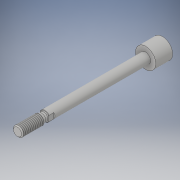
# Autodesk Inventor part: 8112003 DSNU-S-12-30-P---(P)
Saved by Autodesk Inventor 2019 (Build 230136000, 136)
## iProperties
Created: 2023-03-28
Part Number: 8112003 DSNU-S-12-30-P---(P)
Material: Generic
Catalog Web Link: www.cadenas.de
Description: DSNU-S---(P)-ISO cylinder
Vendor: FESTO
Document SubType Name: Modeling
Designer: psAdmin
Manufacturer: FESTO
Mass: 3.24458 g
Surface Area: 20.2529 cm^2
Volume: 3.24458 cm^3
Density: 1 g/cm^3
Appearance: PSOLRGB-175-175-175
Category: PARTsolutions
Company: FESTO
Title: 8112003 DSNU-S-12-30-P
Author: Cadenas PARTsolutions
Comments: ISO cylinder
PSOL_IDENT_0: {$CADENAS_DATA/23d-libs/festo/parts/d/dsnu/parts/dsnu_s_piston.prj},208 {VTYP=3D},{NB=8112003 DSNU-S
PSOL_IDENT_1: -12-30-P---(P)},{LINA=8112003 DSNU-S-12-30-P},{NN=DSNU-S---(P)},{DATE=13.03.2023 13:59:39},{GEOMDATE=
PSOL_IDENT_2: 01.06.2021 09:47:00},{VERSION=},{LINEID=30},{WBVAR=HUB,DA,PE},{WBNUMERIC=HUB}  {NB=8112003 DSNU-S-12
PSOL_IDENT_3: -30-P---(P)},{LINA=8112003 DSNU-S-12-30-P},{KT=DUMMY},{TNR=8112003},{TYP=DSNU-S-12},{KDM=12},{HUB=30
PSOL_IDENT_4: },{DA=P},{DA1='P'},{PE=-},{PE1=},{BWE=-},{BWE1=},{A1=20},{A2=100},{A3=4},{A4=38},{L4=17.000},{AM=16}
PSOL_IDENT_5: ,{B=10},{BE=M10x1},{BEM=10},{BF=8.1},{D1=14},{D4=13.3},{EE=M5},{EEM=5.000},{G=9.65},{G1=11.95},{KK=M
PSOL_IDENT_6: 6},{KKM=6},{KV=14},{KW=4},{L2=75.85},{MM=6},{PL=6.0},{PL1=8.0},{SW=5},{VD=1.5},{WF=13.0},{ZJ=89.30},
PSOL_IDENT_7: {D6=4.8},{AML=14.38},{SWL=3.0},{FDTXF31=3.00},{FDTB31=3.20},{FDTL=70.000}
NB: 8112003 DSNU-S-12-30-P---(P)
NN: DSNU-S---(P)
NT: ISO cylinder
NBSYN: $TNR. $TYP.-$HUB.-$DA.$PE1.$BWE1.---(P)
LINA: 8112003 DSNU-S-12-30-P
CATALOG: Festo
TNR: 8112003
TYP: DSNU-S-12
KDM: 12
HUB: 30
DA: P
DA1: 'P'
PE: -
BWE: -
A1: 20
A2: 100
A3: 4
A4: 38
L4: 17
AM: 16
B: 10
BE: M10x1
BEM: 10
BF: 8.1
D1: 14
D4: 13.3
EE: M5
EEM: 5
KK: M6
KKM: 6
KV: 14
KW: 4
MM: 6
PL: 6
PL1: 8
SW: 5
VD: 1.5
WF: 13
D6: 4.8
AML: 14.38
SWL: 3
FDTXF31: 3
FDTB31: 3.2
SUPPLIER: FESTO
ARTICLENO: 8112003 DSNU-S-12-30-P---(P)
BOMINFO: 8112003 DSNU-S-12-30-P
CREATOR: CADENAS GmbH
Autodesk Inventor part; units mm, degrees
sketch "Sketch_3" plane through (0, 0, 0) normal (1, 0, 0) x (0, 1, 0)
  line L0 (0, 0) -> (0, 86)
  line L1 (0, 86) -> (2.3865, 86)
  line L2 (2.3865, 86) -> (3, 85.3865)
  line L3 (3, 85.3865) -> (3, 73.2685)
  line L4 (3, 73.2685) -> (2.4, 71.62)
  line L5 (2.4, 71.62) -> (2.4, 70.4)
  arc A0 (2.4, 70.4) -> (2.8, 70) centre (2.8, 70.4) ccw
  line L6 (2.8, 70) -> (3, 69.8)
  line L7 (3, 69.8) -> (3, 10)
  line L8 (3, 10) -> (6, 10)
  line L9 (6, 10) -> (6, 0)
  line L10 (6, 0) -> (0, 0)
  line L11 (0, 0) -> (0, 86)
  constraints: 24 end point, 2 point on circle, 1 centre point
revolve "Revolution1" add sketch "Sketch_3" angle 360 about axis through (0, 0, 0) along (0, 0, -1)
thread "Thread1" size "M6x1" class "6g" standard "ISO Metric profile" full length
sketch "Sketch_4" plane through (0, 0, 0) normal (0, 1, 0) x (-1, 0, 0)
  line L0 (5, 65.5566) -> (5, 71)
  line L1 (5, 71) -> (2.5, 71)
  line L2 (2.5, 71) -> (2.5, 67)
  line L3 (2.5, 67) -> (5, 65.5566)
  constraints: 8 end point
extrude "Extrusion1" cut sketch "Sketch_4" along normal mid plane 6
sketch "Sketch_5" plane through (0, 0, 0) normal (0, 1, 0) x (-1, 0, 0)
  line L0 (-2.5, 67) -> (-2.5, 71)
  line L1 (-2.5, 71) -> (-5, 71)
  line L2 (-5, 71) -> (-5, 65.5566)
  line L3 (-5, 65.5566) -> (-2.5, 67)
  constraints: 8 end point
extrude "Extrusion2" cut sketch "Sketch_5" along normal mid plane 6
ref_plane "ANBAU_XY" through (0, 0, 0) normal (0, 0, -1) x (1, 0, 0)
ref_plane "ANBAU_YZ" through (0, 0, 0) normal (1, 0, 0) x (0, -1, 0)
ref_plane "ANBAU_ZX" through (0, 0, 0) normal (0, -1, 0) x (0, 0, -1)
ref_plane "FDT_KSAUFSATZ_XY" through (0, 0, 76.2) normal (0, 0, 1) x (1, 0, 0)
ref_plane "FDT_KSAUFSATZ_YZ" through (0, 0, 76.2) normal (1, 0, 0) x (0, 1, 0)
ref_plane "FDT_KSAUFSATZ_ZX" through (0, 0, 76.2) normal (0, 1, 0) x (0, 0, 1)
ref_plane "FDT_NUT_XY" through (0, 0, 76.2) normal (0, 0, 1) x (1, 0, 0)
ref_plane "FDT_NUT_YZ" through (0, 0, 76.2) normal (1, 0, 0) x (0, 1, 0)
ref_plane "FDT_NUT_ZX" through (0, 0, 76.2) normal (0, 1, 0) x (0, 0, 1)
ref_plane "to_nut_XY" through (0, 0, 83.325) normal (0, 0, 1) x (1, 0, 0)
ref_plane "to_nut_YZ" through (0, 0, 83.325) normal (1, 0, 0) x (0, 1, 0)
ref_plane "to_nut_ZX" through (0, 0, 83.325) normal (0, 1, 0) x (0, 0, 1)
body "Solid1"
